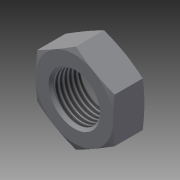
# Autodesk Inventor part: D-9
Saved by Autodesk Inventor 2014 SP2 (Build 180246200, 246)
## iProperties
Created: 2019-01-30
Part Number: D-9
Material: Generic
Catalog Web Link: www.cadenas.de
Description: Mounting Nut for Original Line Cylinders-
Vendor: BIMBA
Document SubType Name: Modeling
Designer: psadmin
Manufacturer: BIMBA
Mass: 3.16349 g
Surface Area: 18.3375 cm^2
Volume: 3.16349 cm^3
Density: 1 g/cm^3
Appearance: PSOLRGB-191-191-191
Category: PARTsolutions
Company: BIMBA
Title: D-9
Author: Cadenas PARTsolutions
PSOL_IDENT_0: {$CADENAS_DATA\23d-libs\bimba\bimba\bimba_imperial\bimba_full_line\original_line_cylinders\accessori
PSOL_IDENT_1: es\mounting_nut.prj},183 {VTYP=3D},{NB=D-9},{LINA=D-9},{NN=Mounting Nut for Original Line Cylinders}
PSOL_IDENT_2: ,{DATE=27.12.2018 09:32:42},{GEOMDATE=10.11.2011 00:00:00},{VERSION=},{LINEID=50},{WBVAR=MAT},{WBNUM
PSOL_IDENT_3: ERIC=}  {NB=D-9},{LINA=D-9},{KT=DUMMY},{PN=D-9},{PN1=D-9},{C=5/8-18},{TH=UNF},{MAT=},{MAT1='','Zinc-
PSOL_IDENT_4: Plated Carbon Steel', '-SS', 'Stainless Steel'},{A=0.94},{A1=0.94000000},{B=0.38},{B1=0.38000000},{N
PSOL_IDENT_5: DM=0.62500000},{PITCH=0.0556},{DIA=-},{DIA2=-},{DIA3=-},{DIA1=0},{DIA4=0.00000000},{DIA5=0.00000000}
PSOL_IDENT_6: ,{T=-},{T2=-},{T3=-},{T1=0},{T4=0.00000000},{T5=0.00000000},{COLOR=0.75,0.75,0.75,0.00},{TT=0.050000
PSOL_IDENT_7: 00},{TO=0.20000000},{PRA=1}
NN: Mounting Nut for Original Line Cylinders
NB: D-9
NBSYN: $PN.
LINA: D-9
PN: D-9
C: 5/8-18
MAT: Zinc-Plated Carbon Steel
A: 0.94
B: 0.38
DIA: -
T: -
SUPPLIER: BIMBA
ARTICLENO: D-9
BOMINFO: D-9
CREATOR: CADENAS GmbH
Autodesk Inventor part; units mm, degrees
sketch "Sketch_8" plane through (0, 0, 0) normal (1, 0, 0) x (0, 1, 0)
  line L0 (0, -9.652) -> (0, 0)
  line L1 (0, 0) -> (11.938, 0)
  line L2 (11.938, 0) -> (14.3256, -0.6398)
  line L3 (14.3256, -0.6398) -> (14.3256, -9.0122)
  line L4 (14.3256, -9.0122) -> (11.938, -9.652)
  line L5 (11.938, -9.652) -> (0, -9.652)
  line L6 (0, -9.652) -> (0, 0)
  constraints: 14 end point
sketch "Sketch_10" plane through (0, 0, 0) normal (0, 0, 1) x (1, 0, 0)
  line L0 (-23.876, -23.876) -> (23.876, -23.876)
  line L1 (23.876, -23.876) -> (23.876, 23.876)
  line L2 (23.876, 23.876) -> (-23.876, 23.876)
  line L3 (-23.876, 23.876) -> (-23.876, -23.876)
  line L4 (-11.938, -6.8924) -> (0, -13.7848)
  line L5 (0, -13.7848) -> (11.938, -6.8924)
  line L6 (11.938, -6.8924) -> (11.938, 6.8924)
  line L7 (11.938, 6.8924) -> (0, 13.7848)
  line L8 (0, 13.7848) -> (-11.938, 6.8924)
  line L9 (-11.938, 6.8924) -> (-11.938, -6.8924)
  constraints: 20 end point
revolve "Revolution1" add sketch "Sketch_8" angle 360 about axis through (0, 0, -9.652) along (0, 0, -1)
extrude "Extrusion1" cut sketch "Sketch_10" against normal blind 9.652
sketch "Sketch_11" plane through (0, 0, 0) normal (1, 0, 0) x (0, 1, 0)
  line L0 (0, -9.652) -> (0, 0)
  line L1 (0, 0) -> (7.9375, 0)
  line L2 (7.9375, 0) -> (7.1742, -0.7633)
  line L3 (7.1742, -0.7633) -> (7.1742, -8.8887)
  line L4 (7.1742, -8.8887) -> (7.9375, -9.652)
  line L5 (7.9375, -9.652) -> (0, -9.652)
  line L6 (0, -9.652) -> (0, 0)
  constraints: 14 end point
revolve "Revolution2" cut sketch "Sketch_11" angle 360 about axis through (0, 0, -9.652) along (0, 0, -1)
thread "Thread1" size "5/8-18 UNF" class "2B" standard "ANSI Unified Screw Threads" full length
ref_plane "NUT_XY" through (0, 0, 0) normal (0, 0, 1) x (1, 0, 0)
ref_plane "NUT_YZ" through (0, 0, 0) normal (1, 0, 0) x (0, 1, 0)
ref_plane "NUT_ZX" through (0, 0, 0) normal (0, 1, 0) x (0, 0, 1)
ref_plane "a1_XY" through (-11.938, 11.938, 0) normal (0, 0, 1) x (1, 0, 0)
ref_plane "a1_YZ" through (-11.938, 11.938, 0) normal (1, 0, 0) x (0, 1, 0)
ref_plane "a1_ZX" through (-11.938, 11.938, 0) normal (0, 1, 0) x (0, 0, 1)
ref_plane "a2_XY" through (11.938, 11.938, 0) normal (0, 0, 1) x (1, 0, 0)
ref_plane "a2_YZ" through (11.938, 11.938, 0) normal (1, 0, 0) x (0, 1, 0)
ref_plane "a2_ZX" through (11.938, 11.938, 0) normal (0, 1, 0) x (0, 0, 1)
ref_plane "b1_XY" through (0, 11.938, 0) normal (1, 0, 0) x (0, 0, -1)
ref_plane "b1_YZ" through (0, 11.938, 0) normal (0, 0, -1) x (0, 1, 0)
ref_plane "b1_ZX" through (0, 11.938, 0) normal (0, 1, 0) x (1, 0, 0)
ref_plane "b2_XY" through (0, 11.938, -9.652) normal (1, 0, 0) x (0, 0, -1)
ref_plane "b2_YZ" through (0, 11.938, -9.652) normal (0, 0, -1) x (0, 1, 0)
ref_plane "b2_ZX" through (0, 11.938, -9.652) normal (0, 1, 0) x (1, 0, 0)
ref_plane "e_XY" through (0, 0, -9.652) normal (1, 0, 0) x (0, 0, -1)
ref_plane "e_YZ" through (0, 0, -9.652) normal (0, 0, -1) x (0, 1, 0)
ref_plane "e_ZX" through (0, 0, -9.652) normal (0, 1, 0) x (1, 0, 0)
ref_plane "ol1_XY" through (0, 0, -11.938) normal (0, 1, 0) x (1, 0, 0)
ref_plane "ol1_YZ" through (0, 0, -11.938) normal (1, 0, 0) x (0, 0, -1)
ref_plane "ol1_ZX" through (0, 0, -11.938) normal (0, 0, -1) x (0, 1, 0)
ref_plane "ol2_XY" through (9.652, 0, -11.938) normal (0, 1, 0) x (1, 0, 0)
ref_plane "ol2_YZ" through (9.652, 0, -11.938) normal (1, 0, 0) x (0, 0, -1)
ref_plane "ol2_ZX" through (9.652, 0, -11.938) normal (0, 0, -1) x (0, 1, 0)
ref_plane "th1_XY" through (0, 7.9375, -9.652) normal (1, 0, 0) x (0, 0, -1)
ref_plane "th1_YZ" through (0, 7.9375, -9.652) normal (0, 0, -1) x (0, 1, 0)
ref_plane "th1_ZX" through (0, 7.9375, -9.652) normal (0, 1, 0) x (1, 0, 0)
ref_plane "th2_XY" through (0, -7.9375, -9.652) normal (1, 0, 0) x (0, 0, -1)
ref_plane "th2_YZ" through (0, -7.9375, -9.652) normal (0, 0, -1) x (0, 1, 0)
ref_plane "th2_ZX" through (0, -7.9375, -9.652) normal (0, 1, 0) x (1, 0, 0)
body "Solid1"
